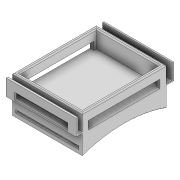
# Autodesk Inventor part: wear1
Saved by Autodesk Inventor 2022 (Build 260153000, 153)
## iProperties
Created: 2021-06-28
Part Number: wear1
Material: Generic
Document SubType Name: Modeling
Designer: Prajwal Patil
Density: 1 g/cm^3
Appearance: Default
Author: Prajwal Patil
Autodesk Inventor part; units mm, degrees
ref_plane "YZ Plane" through (0, 0, 0) normal (1, 0, 0) x (0, 1, 0)
ref_plane "XZ Plane" through (0, 0, 0) normal (0, 1, 0) x (-1, 0, 0)
ref_plane "XY Plane" through (0, 0, 0) normal (0, 0, 1) x (1, 0, 0)
sketch "Sketch1" plane through (0, 0, 0) normal (0, 1, 0) x (-1, 0, 0)
  line L0 (28.4151, 25.1868) -> (-18.6648, 25.1868)
  line L1 (-18.6648, 25.1868) -> (-18.6648, -31.4933)
  line L2 (-18.6648, -31.4933) -> (28.4151, -31.4933)
  line L3 (28.4151, -31.4933) -> (28.4151, 25.1868)
  dimension "d1" = 47.0799
  dimension "d2" = 56.6801
  constraints: 8 end point, 2 parallel, 1 horizontal, 1 perpendicular
  measures "d1" distance of L2.end L1.end
  measures "d2" distance of L1.end L0.end
extrude "Extrusion1" add sketch "Sketch1" along normal blind 15.24
sketch "Sketch3" plane through (18.6648, 0, 25.1868) normal (1, 0, 0) x (0, 0, -1)
  line L0 (0, 15.24) -> (56.6801, 15.24) projected
  line L1 (0, 0) -> (0, 15.24) projected
  line L2 (0, 4.3509) -> (0, 0)
  line L3 (0, 0) -> (56.6801, 0) projected
  line L4 (0, 0) -> (56.6801, 0)
  line L5 (56.6801, 0) -> (56.6801, 4.3509)
  line L6 (56.6801, 0) -> (56.6801, 15.24) projected
  arc A0 (56.6801, 4.3509) -> (0, 4.3509) centre (28.3401, -74.9624) ccw
  point P0 (25.1868, 0)
  constraints: 6 end point, 2 collinear, 2 point on circle, 2 point on line, 1 centre point
extrude "Extrusion2" cut sketch "Sketch3" against normal through all contours A0 L5 L3 L1
fillet "Fillet1" radius 0.254 4 edges at (18.6648, 9.262, -3.1532) (-4.8752, 4.3509, -31.4933) (-28.4151, 9.262, -3.1532) (-4.8752, 4.3509, 25.1868)
sketch "Sketch4" plane through (0, 15.24, 0) normal (0, 1, 0) x (1, 0, 0)
  point P0 (0, 0)
ref_plane "Work Plane1" through (0, 15.24, 0) normal (0, 1, 0) x (1, 0, 0)
sketch "Sketch8" plane through (0, 15.24, 0) normal (0, 1, 0) x (1, 0, 0)
  line L0 (-28.4151, -25.1868) -> (18.6648, -25.1868) projected
  line L1 (-28.4151, -25.1868) -> (18.6648, -25.1868)
  line L2 (18.6648, -25.1868) -> (18.6648, 31.4933)
  line L3 (18.6648, 31.4933) -> (-28.4151, 31.4933)
  line L4 (-28.4151, 31.4933) -> (-28.4151, -25.1868)
  point P0 (0, 0)
  constraints: 8 end point, 2 parallel, 1 horizontal, 1 perpendicular
extrude "Extrusion5" add sketch "Sketch8" along normal blind 14.19
sketch "Sketch9" plane through (0, 29.43, 0) normal (0, 1, 0) x (1, 0, 0)
  line L0 (-28.4151, -25.1868) -> (-28.4151, -25.1722) projected
  line L1 (18.6648, 31.4933) -> (18.6648, 31.4787) projected
  line L2 (18.6648, -25.1722) -> (18.6648, -25.1868) projected
  line L3 (-28.4151, 31.4933) -> (18.6648, 31.4933) projected
  line L4 (-25.8751, -22.6468) -> (16.1248, -22.6468)
  line L5 (16.1248, -22.6468) -> (16.1248, 28.9532)
  line L6 (16.1248, 28.9532) -> (-25.8751, 28.9532)
  line L7 (-25.8751, 28.9532) -> (-25.8751, -22.6468)
  line L8 (-25.8751, -22.6468) -> (16.1248, 28.9532) construction
  line L9 (16.1248, -22.6468) -> (-25.8751, 28.9532) construction
  point P0 (0, 0)
  point P1 (-4.8752, 3.1532)
  dimension "d30" = 41.9999
  dimension "d31" = 51.6
  constraints: 12 end point, 2 midpoint, 2 parallel, 1 horizontal, 1 perpendicular
  measures "d30" distance of L6.end L5.end
  measures "d31" distance of L5.end L4.end
extrude "Extrusion6" cut sketch "Sketch9" against normal blind 11.65
fillet "Fillet2" radius 0.762 4 edges at (-28.4151, 29.43, -3.1532) (-4.8752, 29.43, -31.4933) (18.6648, 29.43, -3.1532) (-4.8752, 29.43, 25.1868)
chamfer "Chamfer3" distance 0.762 angle 45 4 edges at (-4.8752, 29.43, 22.6468) (16.1248, 29.43, -3.1532) (-4.8752, 29.43, -28.9532) (-25.8751, 29.43, -3.1532)
sketch "Sketch10" plane through (18.6648, -74.9624, -3.1532) normal (1, 0, 0) x (0, 0, -1)
  arc A0 (28.3255, 79.5882) -> (-28.3255, 79.5882) centre (0, 0) ccw projected
  line L0 (28.34, 79.673) -> (28.34, 103.6304) projected
  line L1 (-28.3255, 79.5882) -> (28.34, 79.5882)
  line L2 (28.34, 79.5882) -> (28.34, 83.3201)
  line L3 (28.34, 83.3201) -> (-28.3255, 83.3201)
  line L4 (-28.3255, 83.3201) -> (-28.3255, 79.5882)
  point P0 (-3.1532, 74.9624)
  constraints: 8 end point, 2 parallel, 1 horizontal, 1 perpendicular, 1 point on line
ref_plane "Work Plane2" through (18.6648, 4.7106, -31.4933) normal (0, 0, -1) x (-1, 0, 0)
sketch "Sketch11" plane through (18.6648, 4.7106, -31.4933) normal (0, 0, -1) x (-1, 0, 0)
  line L0 (0, 4.8055) -> (0, -0.0848) projected
  line L1 (47.0799, -0.0848) -> (47.0799, 4.8055) projected
  line L2 (0, 4.8055) -> (47.0799, 4.8055)
  line L3 (47.0799, 4.8055) -> (47.0799, -0.0848)
  line L4 (47.0799, -0.0848) -> (0, -0.0848)
  line L5 (0, -0.0848) -> (0, 4.8055)
  line L6 (0.254, 4.5515) -> (46.8259, 4.5515) projected
  line L7 (2.1582, 4.5515) -> (44.8203, 4.5515)
  line L8 (44.8203, 4.5515) -> (44.8203, 2.5848)
  line L9 (44.8203, 2.5848) -> (2.1582, 2.5848)
  line L10 (2.1582, 2.5848) -> (2.1582, 4.5515)
  point P0 (18.6648, -4.7106)
  constraints: 16 end point, 4 parallel, 2 horizontal, 2 perpendicular, 1 point on line
extrude "Extrusion7" cut sketch "Sketch11" against normal through all contours L6 L8 L9 L10
sketch "Sketch15" plane through (18.6648, -74.9624, -3.1532) normal (1, 0, 0) x (0, 0, -1)
  line L0 (-25.8, 92.7424) -> (25.8, 92.7424) projected
  line L1 (-24.298, 98.2163) -> (24.0484, 98.2163)
  line L2 (24.0484, 98.2163) -> (24.0484, 92.7424)
  line L3 (24.0484, 92.7424) -> (-24.298, 92.7424)
  line L4 (-24.298, 92.7424) -> (-24.298, 98.2163)
  point P0 (-3.1532, 74.9624)
  point P1 (-24.298, 92.7424)
  constraints: 8 end point, 2 parallel, 1 horizontal, 1 perpendicular, 1 point on line
extrude "Extrusion8" cut sketch "Sketch15" against normal through all
sketch "Sketch16" plane through (-28.4151, -74.9624, -3.1532) normal (-1, 0, 0) x (0, 0, 1)
  line L0 (28.34, 79.673) -> (28.34, 103.6304) projected
  line L1 (28.34, 92.7388) -> (32.5027, 92.7388)
  line L2 (32.5027, 92.7388) -> (32.5027, 103.6304)
  line L3 (32.5027, 103.6304) -> (28.34, 103.6304)
  line L4 (28.34, 103.6304) -> (28.34, 92.7388)
  point P0 (3.1532, 74.9624)
  constraints: 8 end point, 2 parallel, 1 horizontal, 1 perpendicular, 1 point on line
extrude "Extrusion9" add sketch "Sketch16" against normal blind 47.0799
sketch "Sketch17" plane through (-28.4151, -74.9624, -3.1532) normal (-1, 0, 0) x (0, 0, 1)
  line L0 (32.5027, 103.6304) -> (28.34, 103.6304) projected
  line L1 (28.34, 103.6304) -> (31.2211, 103.6304)
  line L2 (31.2211, 103.6304) -> (31.2211, 93.7101)
  line L3 (31.2211, 93.7101) -> (28.34, 93.7101)
  line L4 (28.34, 93.7101) -> (28.34, 103.6304)
  point P0 (3.1532, 74.9624)
  point P1 (31.2211, 103.6304)
  constraints: 8 end point, 2 parallel, 1 horizontal, 1 perpendicular
extrude "Extrusion10" cut sketch "Sketch17" against normal blind 47.0799
sketch "Sketch18" plane through (18.6648, -74.9624, -3.1532) normal (1, 0, 0) x (0, 0, -1)
  line L0 (28.34, 79.673) -> (28.34, 103.6304) projected
  line L1 (28.34, 103.6304) -> (33.459, 103.6304)
  line L2 (33.459, 103.6304) -> (33.459, 92.5316)
  line L3 (33.459, 92.5316) -> (28.34, 92.5316)
  line L4 (28.34, 92.5316) -> (28.34, 103.6304)
  point P0 (-3.1532, 74.9624)
  constraints: 8 end point, 2 parallel, 1 horizontal, 1 perpendicular
extrude "Extrusion11" add sketch "Sketch18" against normal blind 47.0799
sketch "Sketch19" plane through (18.6648, -74.9624, -3.1532) normal (1, 0, 0) x (0, 0, -1)
  line L0 (28.34, 103.6304) -> (32.4698, 103.6304)
  line L1 (32.4698, 103.6304) -> (32.4698, 93.2696)
  line L2 (32.4698, 93.2696) -> (28.34, 93.2696)
  line L3 (28.34, 93.2696) -> (28.34, 103.6304)
  point P0 (-3.1532, 74.9624)
  constraints: 8 end point, 2 parallel, 1 horizontal, 1 perpendicular
extrude "Extrusion12" cut sketch "Sketch19" against normal blind 47.0799
sketch "Sketch20" plane through (18.6648, 17.5691, -36.6123) normal (0, 0, -1) x (-1, 0, 0)
  line L0 (47.0799, 1.1785) -> (0, 1.1785) projected
  line L1 (5.5367, 5.6549) -> (41.372, 5.6549)
  line L2 (41.372, 5.6549) -> (41.372, 1.1785)
  line L3 (41.372, 1.1785) -> (5.5367, 1.1785)
  line L4 (5.5367, 1.1785) -> (5.5367, 5.6549)
  point P0 (18.6648, -17.5691)
  point P1 (5.5367, 1.1785)
  constraints: 8 end point, 2 parallel, 1 horizontal, 1 perpendicular, 1 point on line
extrude "Extrusion13" cut sketch "Sketch20" against normal blind 1.778
sketch "Sketch21" plane through (-28.4151, 17.7764, 29.3495) normal (0, 0, 1) x (1, 0, 0)
  line L0 (5.7079, 0.9713) -> (5.7079, 5.4477) projected
  line L1 (41.5432, 0.9713) -> (5.7079, 0.9713) projected
  line L2 (5.7079, 5.4477) -> (41.5432, 5.4477)
  line L3 (41.5432, 5.4477) -> (41.5432, 0.9713)
  line L4 (41.5432, 0.9713) -> (5.7079, 0.9713)
  line L5 (5.7079, 0.9713) -> (5.7079, 5.4477)
  point P0 (28.4151, -17.7764)
  constraints: 8 end point, 2 parallel, 1 horizontal, 1 perpendicular
extrude "Extrusion14" cut sketch "Sketch21" against normal blind 1.778
body "Solid1"
